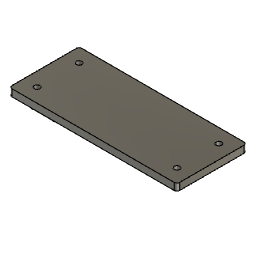
Test v1 (Autodesk Fusion 360 design; units mm, degrees)
Autodesk Fusion 360 part; units mm, degrees
sketch "Sketch1" plane through (0, 0, 0) normal (0, 0, 1) x (1, 0, 0)
  line L0 (0, 0) -> (100, 0)
  line L1 (100, 0) -> (100, 30)
  line L2 (100, 30) -> (0, 30)
  line L3 (0, 30) -> (0, 0)
  line L4 (110, -10) -> (110, 40)
  line L5 (110, 40) -> (-10, 40)
  line L6 (-10, 40) -> (-10, -10)
  line L7 (-10, -10) -> (110, -10)
  circle A0 centre (100, 30) radius 2
  circle A1 centre (100, 0) radius 2
  circle A2 centre (0, 0) radius 2
  circle A3 centre (0, 30) radius 2
  dimension "d1" = 30
  dimension "d2" = 100
  dimension "d3" = 10
  dimension "d4" = 4
  dimension "d5" = 4
  dimension "d6" = 4
  dimension "d7" = 4
  constraint horizontal L0
  constraint vertical L1
  constraint horizontal L2
  constraint vertical L3
  constraint coincident L0.start L3.end
  constraint coincident L1.end L2.start
  constraint coincident L0.end L1.start
  constraint coincident L2.end L3.start
  measures "d1" distance of L0.start L2.end
  measures "d2" distance of L0.start L0.end
  measures "d4" diameter of A0
  measures "d5" diameter of A1
  measures "d6" diameter of A2
  measures "d7" diameter of A3
extrude "Extrude1" add sketch "Sketch1" along normal blind 5 contours L0 L1 L2 L3 A0 A1 A2 A3 | L4 L5 L6 L7 makes body 1
fillet "Fillet1" radius 2 1 edges at (110, -10, 2.5) on bodies 1
fillet "Fillet2" radius 2 1 edges at (110, 40, 2.5) on bodies 1
fillet "Fillet3" radius 2 1 edges at (-10, 40, 2.5) on bodies 1
fillet "Fillet4" radius 2 1 edges at (-10, -10, 2.5) on bodies 1
sketch "Sketch2" plane through (0, 0, 0) normal (0, 1, 0) x (1, 0, 0)
  circle A0 centre (-1, 10) radius 1.95
  dimension "d14" = 3.9
  measures "d14" diameter of A0
extrude "Extrude2" add sketch "Sketch2" along normal blind 15 separate body makes body 2
move_body "Move1" bodies 2 to x (1, 0, 0) y (0, 1, 0) z (0, 0, 1) at (0, -5, -5)
move_body "Move2" bodies 2 to x (0, 0.965926, 0.258819) y (1, 0, 0) z (0, 0.258819, -0.965926) at (2.05, 5.6096, -22.8991)
move_body "Move3" bodies 2 to x (1, 0, 0) y (0, 0.707107, -0.707107) z (0, 0.707107, 0.707107) at (0, 6.3529, -2.0007)
sketch "Sketch3" plane through (0, 0, 0) normal (0, 0, 1) x (1, 0, 0)
